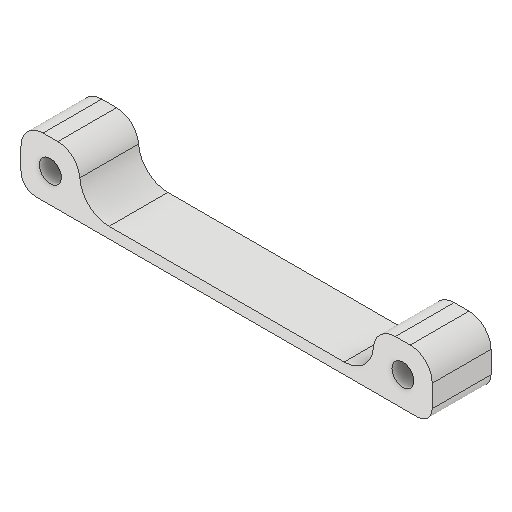
# Autodesk Inventor part: 3DP_ABS_Bowl_Spring
Saved by Autodesk Inventor 2026.1 (Build 301233000, 233)
## iProperties
Created: 2018-05-26
Part Number: 3DP_ABS_Bowl_Spring
Material: ABS Plastic
Document SubType Name: Modeling
Designer: Andrzej
Density: 1.06 g/cm^3
Appearance: Smooth - White
Mass: 1.34192 g
Surface Area: 15.0928 cm^2
Volume: 1.34192 cm^3
Author: Andrzej
Autodesk Inventor part; units mm, degrees
ref_plane "YZ Plane" through (0, 0, 0) normal (1, 0, 0) x (0, 1, 0)
ref_plane "XZ Plane" through (0, 0, 0) normal (0, 1, 0) x (-1, 0, 0)
ref_plane "XY Plane" through (0, 0, 0) normal (0, 0, 1) x (1, 0, 0)
sketch "Sketch1" plane through (0, 0, 0) normal (0, 0, 1) x (1, 0, 0)
  line L0 (-3.4439, 0.5518) -> (36.5561, 0.5518)
  line L1 (44.5561, -0.9482) -> (-11.4439, -0.9482)
  line L2 (-3.4439, 0.5518) -> (-3.4439, 7.0518)
  line L3 (-3.4439, 7.0518) -> (-11.4439, 7.0518)
  line L4 (36.5561, 0.5518) -> (36.5561, 7.0518)
  line L5 (36.5561, 7.0518) -> (44.5561, 7.0518)
  line L6 (-11.4439, 7.0518) -> (-11.4439, -0.9482)
  line L7 (44.5561, 7.0518) -> (44.5561, -0.9482)
  point P0 (0, 0)
  point P1 (-7.4439, 3.0518)
  point P2 (40.5561, 3.0518)
  dimension "d2" = 8
  dimension "d4" = 8
  dimension "d5" = 1.5
  dimension "d6" = 56
  dimension "d7" = 8
  dimension "d8" = 8
  dimension "d9" = 4
  dimension "d10" = 4
  dimension "d11" = 4
  dimension "d12" = 4
  constraints: 16 end point, 2 parallel, 1 horizontal, 1 perpendicular
  measures "d2" distance of L3.end L2.end
  measures "d4" distance of L4.end L5.end
  measures "d5" distance between parallel lines of L1 L0
  measures "d6" distance between parallel lines of L7 L6
  measures "d7" distance between parallel lines of L1 L3
  measures "d8" distance of L5.end L1.start
  measures "d9" distance from line of L3 point (-7.444, 3.052)
  measures "d10" distance from line of L6 point (-7.444, 3.052)
  measures "d11" distance from line of L5 point (40.556, 3.052)
  measures "d12" distance from line of L7 point (40.556, 3.052)
extrude "Extrusion1" add sketch "Sketch1" along normal blind 8
hole "Hole1" at (40.5561, 3.0518, 0) at (-7.4439, 3.0518, 0) direction (0, 0, 1) diameter 3 end through all
fillet "Fillet1" radius 4 2 edges at (-3.4439, 0.5518, 4) (36.5561, 0.5518, 4)
fillet "Fillet2" radius 3 4 edges at (-3.4439, 7.0518, 4) (-11.4439, 7.0518, 4) (44.5561, 7.0518, 4) (36.5561, 7.0518, 4)
fillet "Fillet3" radius 2 2 edges at (44.5561, -0.9482, 4) (-11.4439, -0.9482, 4)
equation "\"d4\" = d2"
equation "\"d7\" = d2"
equation "\"d8\" = d2"
equation "\"d9\" = 0.5 * d2"
equation "\"d10\" = 0.5 * d2"
equation "\"d11\" = 0.5 * d2"
equation "\"d12\" = 0.5 * d2"
body "Solid1"
